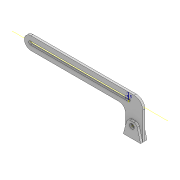
# Autodesk Inventor part: Bancada
Saved by Autodesk Inventor 2021 (Build 250183000, 183)
## iProperties
Created: 2021-07-04
Part Number: Bancada
Material: Generic
Document SubType Name: Modeling
Designer: Santiago
Density: 1 g/cm^3
Appearance: Default
Author: Santiago
Autodesk Inventor part; units mm, degrees
ref_plane "YZ Plane" through (0, 0, 0) normal (1, 0, 0) x (0, 1, 0)
ref_plane "XZ Plane" through (0, 0, 0) normal (0, 1, 0) x (-1, 0, 0)
ref_plane "XY Plane" through (0, 0, 0) normal (0, 0, 1) x (1, 0, 0)
sketch "Sketch1" plane through (0, 0, 0) normal (0, 0, 1) x (1, 0, 0)
  line L0 (0, 0) -> (20, 0)
  line L1 (0, 0) -> (-20, 0)
  line L2 (-20, 0) -> (-12.2354, 28.9778)
  line L3 (0, 0) -> (0, 49.8144) construction
  line L4 (20, 0) -> (12.2354, 28.9778)
  line L5 (-4.508, 34.9072) -> (4.508, 34.9072)
  arc A0 (-4.508, 34.9072) -> (-12.2354, 28.9778) centre (-4.508, 26.9072) ccw
  arc A1 (12.2354, 28.9778) -> (4.508, 34.9072) centre (4.508, 26.9072) ccw
  circle A2 centre (0, 24.9072) radius 5.6106
  line L6 (0, 24.9072) -> (0, 69.9072) construction
  line L7 (0, 69.9072) -> (-240.8319, 69.9072) construction
  line L8 (-240.8319, 69.9072) -> (0, 24.9072) construction
  point P0 (-10.6466, 34.9072)
  point P1 (10.6466, 34.9072)
  dimension "d0" = 20
  dimension "d1" = 20
  dimension "d2" = 75
  dimension "d3" = 8
  dimension "d4" = 8
  dimension "d8" = 30
  dimension "d16" = 45
  dimension "d17" = 10
  dimension "d18" = 245
  constraints: 18 end point, 5 point on line, 4 horizontal, 4 point on circle, 4 tangent, 3 centre point, 1 midpoint, 1 symmetric about line, 1 vertical
  measures "d0" distance of L0.start L0.end
  measures "d1" distance of L0.start L1.end
  measures "d2" angle of L1 L2
  measures "d3" radius of A0
  measures "d4" radius of A1
  measures "d8" distance of L1.end L2.end
  measures "d16" distance of L6.start L6.end
  measures "d17" distance from line of L6.start L5
  measures "d18" distance of L7.end L6.start
extrude "Extrusion2" add sketch "Sketch1" along normal blind 15
sketch "Sketch3" plane through (-4.508, 34.9072, 0) normal (0, 1, 0) x (1, 0, 0)
  line L0 (-15.492, -15) -> (24.508, -15) projected
  line L1 (4.508, -15) -> (4.508, 0)
  line L2 (4.508, 0) -> (4.508, -7.5)
  line L3 (24.508, 0) -> (24.508, -15) projected
  line L4 (-15.492, -5) -> (24.508, -5)
  line L5 (24.508, -5) -> (24.508, -10)
  line L6 (24.508, -10) -> (-15.492, -10)
  line L7 (-15.492, -10) -> (-15.492, -5)
  line L8 (-15.492, -5) -> (24.508, -10) construction
  line L9 (24.508, -5) -> (-15.492, -10) construction
  point P0 (24.508, -5)
  dimension "d11" = 5
  constraints: 16 end point, 4 midpoint, 2 parallel, 1 horizontal, 1 perpendicular, 1 point on line, 1 vertical
  measures "d11" distance of L4.end L5.end
extrude "Extrusion3" add sketch "Sketch3" along normal blind 50 and the other way blind 34.907 contours L6 L7 L4 L1 | L1 L4 L3 L6
sketch "Sketch6" plane through (-20, 0.0002, 10) normal (-1, 0, 0) x (0, 0, 1)
  line L0 (0, 0) -> (0, 84.907) projected
  line L1 (-5, 54.907) -> (0, 54.907)
  line L2 (0, 54.907) -> (0, 84.907)
  line L3 (0, 84.907) -> (-5, 84.907)
  line L4 (-5, 84.907) -> (-5, 54.907)
  line L5 (-5, 54.907) -> (0, 84.907) construction
  line L6 (0, 54.907) -> (-5, 84.907) construction
  point P0 (-10, -0.0002)
  point P1 (-2.5, 69.907)
  point P2 (0, 54.907)
  dimension "d19" = 30
  constraints: 12 end point, 2 midpoint, 2 parallel, 1 horizontal, 1 perpendicular
  measures "d19" distance of L3.end L1.start
extrude "Extrusion4" add sketch "Sketch6" along normal blind 235
fillet "Fillet1" radius 20 1 edges at (20, 84.9072, 7.5)
sketch "Sketch7" plane through (4.508, 34.9072, 5) normal (0, 0, -1) x (-1, 0, 0)
  line L0 (4.508, 35) -> (245.3399, 35) construction
  line L1 (245.3399, 35) -> (17.4625, 35) construction
  line L2 (245.3399, 39) -> (17.4625, 39)
  line L3 (17.4625, 31) -> (245.3399, 31)
  arc A0 (245.3399, 31) -> (245.3399, 39) centre (245.3399, 35) ccw
  arc A1 (17.4625, 39) -> (17.4625, 31) centre (17.4625, 35) ccw
  point P0 (4.508, -34.9072)
  point P1 (131.4012, 35)
  dimension "d25" = 8
  constraints: 8 end point, 4 point on circle, 4 tangent, 2 centre point, 1 midpoint, 1 parallel, 1 point on line
  measures "d25" diameter of A1
fillet "Fillet4" radius 15 2 edges at (-255, 84.9072, 7.5) (-255, 54.9072, 7.5)
fillet "Fillet5" radius 15 1 edges at (-20, 54.9072, 7.5)
extrude "Extrusion5" cut sketch "Sketch7" against normal blind 5
hole "Hole1" at (0, 24.9072, 0) direction (0, 0, 1) diameter 8 end through all
sketch "Sketch8" plane through (0, 0, 15) normal (0, 0, 1) x (1, 0, 0)
  circle A0 centre (0, 24.9072) radius 4 projected
  line L0 (0, 24.9072) -> (0, 69.9072)
  line L1 (-12.9545, 65.9072) -> (-240.8319, 65.9072) projected
  line L2 (0, 24.9072) -> (45, 24.9072) construction
  circle A1 centre (0, 24.9072) radius 5.6106 projected
  arc A2 (-240.8319, 73.9072) -> (-240.8319, 65.9072) centre (-240.8319, 69.9072) ccw projected
  line L3 (0, 24.9072) -> (-240.8319, 69.9072)
  line L4 (-240.8319, 69.9072) -> (0, 69.9072)
  point P0 (0, 0)
  dimension "d37" = 45
  dimension "d38" = 90
  constraints: 8 end point, 2 perpendicular, 1 horizontal
  measures "d37" distance of L0.start L0.end
  measures "d38" angle of L2 L0
ref_plane "Work Plane1" through (-12.953, 0.0002, 10) normal (1, 0, 0) x (0, 0, -1)
sketch "Sketch9" plane through (-12.953, 0.0002, 10) normal (1, 0, 0) x (0, 0, -1)
  line L0 (0, 64.907) -> (0, 84.907) projected
  line L1 (0, 84.907) -> (0, 69.907)
  line L2 (0, 69.907) -> (2.5, 69.907)
  point P0 (10, -0.0002)
  dimension "d40" = 15
  dimension "d41" = 2.5
  constraints: 4 end point, 1 horizontal, 1 point on line
  measures "d40" distance of L0.end L1.end
  measures "d41" distance of L1.end L2.end
body "Solid2"
